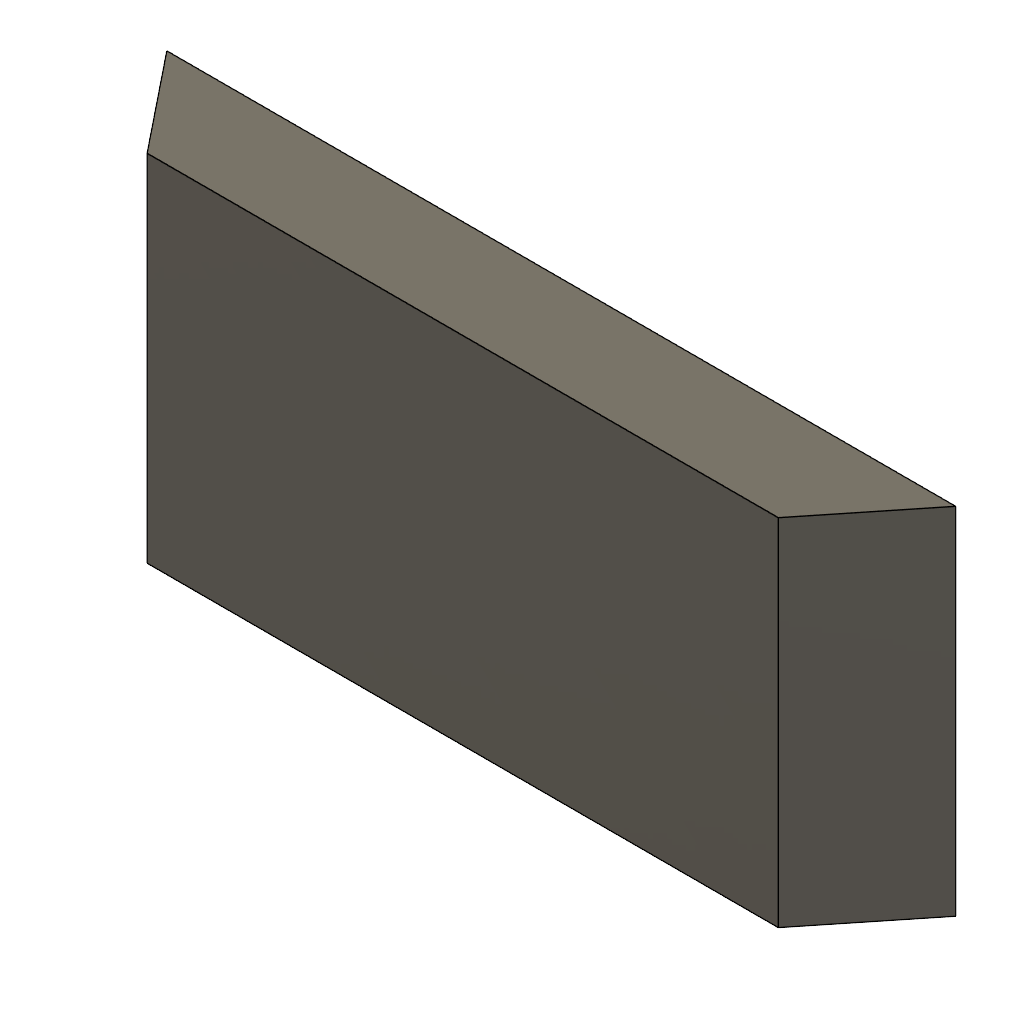
fit_coupon_male (Autodesk Fusion 360 design; units mm, degrees)
part number: 2026-10-03-13-12-52-050
Autodesk Fusion 360 part; units mm, degrees
ref_plane "工作平面1" through (0, 0, 2.3) normal (0, 0, 1) x (1, 0, 0)
sketch "草图1" plane through (0, 0, 2.3) normal (0, 0, 1) x (1, 0, 0)
  line L0 (-20, -9) -> (20, -9)
  line L1 (20, -9) -> (20, 9)
  line L2 (20, 9) -> (-20, 9)
  line L3 (-20, 9) -> (-20, -9)
ref_plane "工作平面2" through (0, 0, 7.3) normal (0, 0, 1) x (1, 0, 0)
sketch "草图2" plane through (0, 0, 7.3) normal (0, 0, 1) x (1, 0, 0)
  line L0 (-16, -9) -> (16, -9)
  line L1 (16, -9) -> (16, 9)
  line L2 (16, 9) -> (-16, 9)
  line L3 (-16, 9) -> (-16, -9)
loft "Coupon male dovetail" add profiles "草图1", "草图2" section 1 section 2
